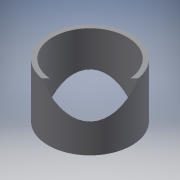
# Autodesk Inventor part: 零件9
Saved by Autodesk Inventor 2016 (Build 200138000, 138)
## iProperties
Created: 2016-12-22
Part Number: 零件9
Material: 一般
Document SubType Name: Modeling
Designer: Alex
Density: 1 g/cm^3
Appearance: 預設
Author: Alex
Autodesk Inventor part; units mm, degrees
ref_plane "YZ Plane" through (0, 0, 0) normal (1, 0, 0) x (0, 1, 0)
ref_plane "XZ Plane" through (0, 0, 0) normal (0, 1, 0) x (-1, 0, 0)
ref_plane "XY Plane" through (0, 0, 0) normal (0, 0, 1) x (1, 0, 0)
sketch "草圖1" plane through (0, 0, 0) normal (0, 0, 1) x (1, 0, 0)
  circle A0 centre (0, 0) radius 25.4
  circle A1 centre (0, 0) radius 22.6806
  dimension "d0" = 50.8
  constraints: 2 centre point, 2 coincident
  measures "d0" diameter of A0
extrude "擠出1" add sketch "草圖1" along normal blind 36
